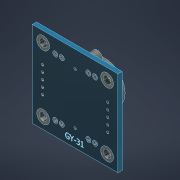
# Autodesk Inventor part: Color_sensor_PCB
Saved by Autodesk Inventor 2021 (Build 250183000, 183)
## iProperties
Created: 2016-09-21
Part Number: Color_sensor_PCB
Material: ABS Plastic
Document SubType Name: Modeling
Designer: Ádi
Density: 1.06 g/cm^3
Appearance: Sky Blue Medium
Author: Ádi
Autodesk Inventor part; units mm, degrees
(part 1 of 2)
ref_plane "YZ Plane" through (0, 0, 0) normal (1, 0, 0) x (0, 1, 0)
ref_plane "XZ Plane" through (0, 0, 0) normal (0, 1, 0) x (-1, 0, 0)
ref_plane "XY Plane" through (0, 0, 0) normal (0, 0, 1) x (1, 0, 0)
sketch "Sketch1" plane through (0, 0, 0) normal (0, 1, 0) x (-1, 0, 0)
  line L0 (-16.75, 16.75) -> (16.75, 16.75)
  line L1 (16.75, 16.75) -> (16.75, -16.75)
  line L2 (16.75, -16.75) -> (-16.75, -16.75)
  line L3 (-16.75, -16.75) -> (-16.75, 16.75)
  line L4 (-16.75, 16.75) -> (16.75, -16.75) construction
  line L5 (16.75, 16.75) -> (-16.75, -16.75) construction
  point P0 (0, 0)
  dimension "d0" = 33.5
  dimension "d1" = 33.5
  constraints: 12 end point, 2 midpoint, 2 parallel, 1 horizontal, 1 perpendicular
  measures "d0" distance of L1.end L2.end
  measures "d1" distance of L0.end L1.end
extrude "Extrusion1" add sketch "Sketch1" along normal blind 1.65
sketch "Sketch2" plane through (0, 1.65, 0) normal (0, 1, 0) x (1, 0, 0)
  line L0 (16.75, -16.75) -> (16.75, 16.75) projected
  line L1 (-16.75, -16.75) -> (16.75, -16.75) projected
  point P0 (0, 0)
  point P1 (-12.4997, -12.6164)
  point P2 (-12.4997, 12.3836)
  point P3 (12.5, 12.5)
  point P4 (12.5, -12.5)
  dimension "d4" = 25
  dimension "d5" = 25
  dimension "d6" = 25
  dimension "d7" = 25
  dimension "d8" = 0
  dimension "d9" = 4.25
  dimension "d10" = 4.25
  measures "d4" distance of point (12.5, 12.5) point (12.5, -12.5)
  measures "d5" distance of point (-12.5, 12.384) point (12.5, 12.5)
  measures "d6" distance of point (-12.5, -12.616) point (-12.5, 12.384)
  measures "d7" distance of point (12.5, -12.5) point (-12.5, -12.616)
  measures "d8" horizontal distance of point (12.5, 12.5) point (12.5, -12.5)
  measures "d9" distance from line of L0 point (12.5, -12.5)
  measures "d10" distance from line of point (12.5, -12.5) L1
hole "Hole1" at (-12.4997, 1.65, 12.6164) at (-12.4997, 1.65, -12.3836) at (12.5, 1.65, -12.5) at (12.5, 1.65, 12.5) direction (0, -1, 0) diameter 3 depth 8 tip angle 118
sketch "Sketch3" plane through (0, 1.65, 0) normal (0, 1, 0) x (1, 0, 0)
  circle A0 centre (12.5, 12.5) radius 1.5 projected
  circle A1 centre (-12.4997, -12.6164) radius 1.5 projected
  circle A2 centre (-12.4997, 12.3836) radius 1.5 projected
  circle A3 centre (12.5, -12.5) radius 1.5 projected
  line L0 (-16.75, -16.75) -> (16.75, -16.75) projected
  line L1 (16.75, -16.75) -> (16.75, 16.75) projected
  line L2 (16.75, 16.75) -> (-16.75, 16.75) projected
  line L3 (-16.75, 16.75) -> (-16.75, -16.75) projected
  circle A4 centre (-12.4997, -12.6164) radius 1.5 projected
  circle A5 centre (-12.4997, -12.6164) radius 2.5
  circle A6 centre (-12.4997, 12.3836) radius 2.5
  circle A7 centre (12.5, 12.5) radius 2.5
  circle A8 centre (12.5, -12.5) radius 1.5 projected
  circle A9 centre (12.5, -12.5) radius 2.5
  point P0 (0, 0)
  dimension "d18" = 5
  dimension "d19" = 5
  dimension "d20" = 5
  dimension "d21" = 5
  constraints: 4 centre point, 4 coincident
  measures "d18" diameter of A5
  measures "d19" diameter of A6
  measures "d20" diameter of A7
  measures "d21" diameter of A9
extrude "Extrusion2" add sketch "Sketch3" along normal blind 0.01 contours A5 | A6 | A7 | A9
sketch "Sketch4" plane through (0, 0, 0) normal (0, -1, 0) x (1, 0, 0)
  circle A0 centre (12.5, -12.5) radius 1.5 projected
  circle A1 centre (-12.4997, 12.6164) radius 1.5 projected
  circle A2 centre (-12.4997, -12.3836) radius 1.5 projected
  circle A3 centre (12.5, 12.5) radius 1.5 projected
  line L0 (16.75, 16.75) -> (-16.75, 16.75) projected
  line L1 (-16.75, 16.75) -> (-16.75, -16.75) projected
  line L2 (-16.75, -16.75) -> (16.75, -16.75) projected
  line L3 (16.75, -16.75) -> (16.75, 16.75) projected
  circle A4 centre (12.5, 12.5) radius 2.5 projected
  circle A5 centre (12.5, 12.5) radius 2.5
  circle A6 centre (12.5, -12.5) radius 2.5
  circle A7 centre (-12.4997, -12.3836) radius 2.5
  circle A8 centre (-12.4997, 12.6164) radius 2.5
  point P0 (0, 0)
  constraints: 4 centre point, 4 coincident
extrude "Extrusion3" add sketch "Sketch4" along normal blind 0.01 contours A4 | A6 | A7 | A8
sketch "Sketch5" plane through (0, 0, 0) normal (0, -1, 0) x (1, 0, 0)
  line L0 (16.75, -16.75) -> (16.75, 16.75) projected
  line L1 (16.75, -16.75) -> (-16.75, -16.75) projected
  point P0 (0, 0)
  point P1 (12.75, -5.07)
  point P2 (12.75, -2.53)
  point P3 (12.75, 0.01)
  point P4 (12.75, 2.55)
  point P5 (12.75, 5.09)
  dimension "d26" = 4
  dimension "d29" = 2.54
  dimension "d41" = 11.68
  constraints: 1 vertical, 4 other
  measures "d26" distance from line of point (12.75, -5.07) L0
  measures "d29" distance of point (12.75, -5.07) point (12.75, -2.53)
  measures "d41" distance from line of L1 point (12.75, -5.07)
hole "Hole2" at (12.75, 0, -5.07) at (12.75, 0, -2.53) at (12.75, 0, 0.01) at (12.75, 0, 2.55) at (12.75, 0, 5.09) direction (0, 1, 0) diameter 1 depth 8 tip angle 118
mirror "Mirror1" about plane through (0, 0, 0) normal (1, 0, 0) of "Hole2"
sketch "Sketch6" plane through (0, 1.65, 0) normal (0, 1, 0) x (1, 0, 0)
  circle A0 centre (-12.75, -2.55) radius 0.5 projected
  circle A1 centre (-12.75, 2.53) radius 0.5 projected
  circle A2 centre (-12.75, 5.07) radius 0.5 projected
  circle A3 centre (-12.75, -0.01) radius 0.5 projected
  circle A4 centre (-12.75, -5.09) radius 0.5 projected
  circle A5 centre (12.75, -2.55) radius 0.5 projected
  circle A6 centre (12.75, 2.53) radius 0.5 projected
  circle A7 centre (12.75, 5.07) radius 0.5 projected
  circle A8 centre (12.75, -0.01) radius 0.5 projected
  circle A9 centre (12.75, -5.09) radius 0.5 projected
  circle A10 centre (12.5, 12.5) radius 2.5 projected
  circle A11 centre (-12.4997, -12.6164) radius 2.5 projected
  circle A12 centre (-12.4997, 12.3836) radius 2.5 projected
  circle A13 centre (12.5, -12.5) radius 2.5 projected
  line L0 (-16.75, -16.75) -> (16.75, -16.75) projected
  line L1 (16.75, -16.75) -> (16.75, 16.75) projected
  line L2 (16.75, 16.75) -> (-16.75, 16.75) projected
  line L3 (-16.75, 16.75) -> (-16.75, -16.75) projected
  circle A14 centre (12.75, 5.07) radius 0.5 projected
  circle A15 centre (12.75, 5.07) radius 1
  circle A16 centre (12.75, 2.53) radius 0.5 projected
  circle A17 centre (12.75, 2.53) radius 1
  circle A18 centre (12.75, -0.01) radius 0.5 projected
  circle A19 centre (12.75, -0.01) radius 1
  circle A20 centre (12.75, -2.55) radius 1
  circle A21 centre (12.75, -5.09) radius 1
  point P0 (0, 0)
  dimension "d42" = 2
  dimension "d43" = 2
  dimension "d44" = 2
  dimension "d45" = 2
  dimension "d46" = 2
  constraints: 5 centre point, 5 coincident
  measures "d42" diameter of A15
  measures "d43" diameter of A17
  measures "d44" diameter of A19
  measures "d45" diameter of A20
  measures "d46" diameter of A21
extrude "Extrusion4" add sketch "Sketch6" along normal blind 0.01 contours A15 | A17 | A19 | A20 | A21
mirror "Mirror2" about plane through (0, 0, 0) normal (1, 0, 0) of "Extrusion4"
sketch "Sketch7" plane through (0, 1.65, 0) normal (0, 1, 0) x (1, 0, 0)
  line L0 (14.4, -6.51) -> (11.1, -6.51)
  line L1 (11.1, -6.51) -> (11.1, 6.49)
  line L2 (11.1, 6.49) -> (14.4, 6.49)
  line L3 (14.4, 6.49) -> (14.4, -6.51)
  circle A0 centre (12.75, -0.01) radius 0.5 projected
  line L4 (14.4, -6.51) -> (11.1, 6.49) construction
  line L5 (11.1, -6.51) -> (14.4, 6.49) construction
  line L6 (14, 6.09) -> (11.5, 6.09)
  line L7 (11.5, 6.09) -> (11.5, -6.11)
  line L8 (11.5, -6.11) -> (14, -6.11)
  line L9 (14, -6.11) -> (14, 6.09)
  line L10 (14, 6.09) -> (11.5, -6.11) construction
  line L11 (11.5, 6.09) -> (14, -6.11) construction
  point P0 (0, 0)
  dimension "d49" = 3.3
  dimension "d50" = 13
  dimension "d51" = 0.4
  dimension "d52" = 0.4
  constraints: 24 end point, 4 midpoint, 4 parallel, 2 horizontal, 2 perpendicular
  measures "d49" distance of L1.end L2.end
  measures "d50" distance between parallel lines of L2 L0
  measures "d51" distance between parallel lines of L8 L0
  measures "d52" distance between parallel lines of L1 L7
extrude "Extrusion5" add sketch "Sketch7" along normal blind 0.01 contours L0 L1 L2 L3
mirror "Mirror3" about plane through (0, 0, 0) normal (1, 0, 0) of "Extrusion5"
sketch "Sketch8" plane through (0, 1.65, 0) normal (0, 1, 0) x (1, 0, 0)
  line L0 (14.9046, -7.6087) -> (14.9046, 13.5384) construction
  line L1 (14.9046, 13.5384) -> (16.4666, 13.5384) construction
  line L2 (16.4666, 13.5384) -> (16.4666, -7.6087) construction
  line L3 (16.4666, -7.6087) -> (14.9046, -7.6087) construction
  line L4 (-14.8755, 8.2478) -> (-14.8755, -7.59) construction
  line L5 (-14.8755, -7.59) -> (-16.1781, -7.59) construction
  line L6 (-16.1781, -7.59) -> (-16.1781, 8.2478) construction
  line L7 (-16.1781, 8.2478) -> (-14.8755, 8.2478) construction
  line L8 (14.93, -6.5754) -> (16.18, -7.0059)
  line L9 (16.18, -7.0059) -> (16.18, -7.1852)
  line L10 (16.18, -7.1852) -> (14.93, -7.6157)
  line L11 (14.93, -7.6157) -> (14.93, -7.4375)
  line L12 (14.93, -7.4375) -> (15.9682, -7.091)
  line L13 (15.9682, -7.091) -> (14.93, -6.7446)
  line L14 (14.93, -6.7446) -> (14.93, -6.5754)
  spline S0 degree 2 poles (16.2022, -5.9677) (16.2022, -6.0892) (16.1202, -6.2948) (16.0381, -6.3698) knots 0 0 0 1 2 2 2
  spline S1 degree 2 poles (16.0381, -6.3698) (15.9571, -6.4448) (15.714, -6.5268) (15.556, -6.5268) knots 0 0 0 1 2 2 2
  spline S2 degree 2 poles (15.556, -6.5268) (15.399, -6.5268) (15.166, -6.4468) (15.0799, -6.3708) knots 0 0 0 1 2 2 2
  spline S3 degree 2 poles (15.0799, -6.3708) (14.9958, -6.2959) (14.9077, -6.0912) (14.9077, -5.9646) knots 0 0 0 1 2 2 2
  spline S4 degree 2 poles (14.9077, -5.9646) (14.9077, -5.9018) (14.9259, -5.7914) (14.9401, -5.7448) knots 0 0 0 1 2 2 2
  spline S5 degree 2 poles (14.9401, -5.7448) (14.9533, -5.7043) (14.9907, -5.6202) (15.013, -5.5787) knots 0 0 0 1 2 2 2
  line L15 (15.013, -5.5787) -> (15.2136, -5.5787)
  line L16 (15.2136, -5.5787) -> (15.2136, -5.5918)
  spline S6 degree 2 poles (15.2136, -5.5918) (15.1933, -5.6141) (15.1366, -5.683) (15.1093, -5.7326) knots 0 0 0 1 2 2 2
  spline S7 degree 2 poles (15.1093, -5.7326) (15.0829, -5.7803) (15.0495, -5.8927) (15.0495, -5.9656) knots 0 0 0 1 2 2 2
  spline S8 degree 2 poles (15.0495, -5.9656) (15.0495, -6.0456) (15.1153, -6.1885) (15.1781, -6.2422) knots 0 0 0 1 2 2 2
  spline S9 degree 2 poles (15.1781, -6.2422) (15.242, -6.2948) (15.4354, -6.3536) (15.556, -6.3536) knots 0 0 0 1 2 2 2
  spline S10 degree 2 poles (15.556, -6.3536) (15.6846, -6.3536) (15.87, -6.2918) (15.9338, -6.2381) knots 0 0 0 1 2 2 2
  spline S11 degree 2 poles (15.9338, -6.2381) (15.9956, -6.1854) (16.0584, -6.0446) (16.0584, -5.9656) knots 0 0 0 1 2 2 2
  spline S12 degree 2 poles (16.0584, -5.9656) (16.0584, -5.8937) (16.0229, -5.7711) (15.9966, -5.7235) knots 0 0 0 1 2 2 2
  spline S13 degree 2 poles (15.9966, -5.7235) (15.9703, -5.6779) (15.9156, -5.6101) (15.8963, -5.5908) knots 0 0 0 1 2 2 2
  line L17 (15.8963, -5.5908) -> (15.8963, -5.5787)
  line L18 (15.8963, -5.5787) -> (16.0949, -5.5787)
  spline S14 degree 2 poles (16.0949, -5.5787) (16.1141, -5.6202) (16.1496, -5.6931) (16.1658, -5.7448) knots 0 0 0 1 2 2 2
  spline S15 degree 2 poles (16.1658, -5.7448) (16.184, -5.7995) (16.2022, -5.8927) (16.2022, -5.9677) knots 0 0 0 1 2 2 2
  spline S16 degree 2 poles (16.2022, -4.9354) (16.2022, -5.057) (16.1202, -5.2626) (16.0381, -5.3376) knots 0 0 0 1 2 2 2
  spline S17 degree 2 poles (16.0381, -5.3376) (15.9571, -5.4125) (15.714, -5.4946) (15.556, -5.4946) knots 0 0 0 1 2 2 2
  spline S18 degree 2 poles (15.556, -5.4946) (15.399, -5.4946) (15.166, -5.4146) (15.0799, -5.3386) knots 0 0 0 1 2 2 2
  spline S19 degree 2 poles (15.0799, -5.3386) (14.9958, -5.2636) (14.9077, -5.059) (14.9077, -4.9324) knots 0 0 0 1 2 2 2
  spline S20 degree 2 poles (14.9077, -4.9324) (14.9077, -4.8696) (14.9259, -4.7592) (14.9401, -4.7126) knots 0 0 0 1 2 2 2
  spline S21 degree 2 poles (14.9401, -4.7126) (14.9533, -4.6721) (14.9907, -4.588) (15.013, -4.5465) knots 0 0 0 1 2 2 2
  line L19 (15.013, -4.5465) -> (15.2136, -4.5465)
  line L20 (15.2136, -4.5465) -> (15.2136, -4.5596)
  spline S22 degree 2 poles (15.2136, -4.5596) (15.1933, -4.5819) (15.1366, -4.6508) (15.1093, -4.7004) knots 0 0 0 1 2 2 2
  spline S23 degree 2 poles (15.1093, -4.7004) (15.0829, -4.748) (15.0495, -4.8605) (15.0495, -4.9334) knots 0 0 0 1 2 2 2
  spline S24 degree 2 poles (15.0495, -4.9334) (15.0495, -5.0134) (15.1153, -5.1563) (15.1781, -5.21) knots 0 0 0 1 2 2 2
  spline S25 degree 2 poles (15.1781, -5.21) (15.242, -5.2626) (15.4354, -5.3214) (15.556, -5.3214) knots 0 0 0 1 2 2 2
  spline S26 degree 2 poles (15.556, -5.3214) (15.6846, -5.3214) (15.87, -5.2596) (15.9338, -5.2059) knots 0 0 0 1 2 2 2
  spline S27 degree 2 poles (15.9338, -5.2059) (15.9956, -5.1532) (16.0584, -5.0124) (16.0584, -4.9334) knots 0 0 0 1 2 2 2
  spline S28 degree 2 poles (16.0584, -4.9334) (16.0584, -4.8615) (16.0229, -4.7389) (15.9966, -4.6913) knots 0 0 0 1 2 2 2
  spline S29 degree 2 poles (15.9966, -4.6913) (15.9703, -4.6457) (15.9156, -4.5779) (15.8963, -4.5586) knots 0 0 0 1 2 2 2
  line L21 (15.8963, -4.5586) -> (15.8963, -4.5465)
  line L22 (15.8963, -4.5465) -> (16.0949, -4.5465)
  spline S30 degree 2 poles (16.0949, -4.5465) (16.1141, -4.588) (16.1496, -4.6609) (16.1658, -4.7126) knots 0 0 0 1 2 2 2
  spline S31 degree 2 poles (16.1658, -4.7126) (16.184, -4.7673) (16.2022, -4.8605) (16.2022, -4.9354) knots 0 0 0 1 2 2 2
  spline S32 degree 2 poles (16.2022, -3.5061) (16.2022, -3.6419) (16.1455, -3.8323) (16.105, -3.9164) knots 0 0 0 1 2 2 2
  line L23 (16.105, -3.9164) -> (15.8963, -3.9164)
  line L24 (15.8963, -3.9164) -> (15.8963, -3.9042)
  spline S33 degree 2 poles (15.8963, -3.9042) (15.9733, -3.8222) (16.0584, -3.6145) (16.0584, -3.5183) knots 0 0 0 1 2 2 2
  spline S34 degree 2 poles (16.0584, -3.5183) (16.0584, -3.3805) (15.9439, -3.2397) (15.8497, -3.2397) knots 0 0 0 1 2 2 2
  spline S35 degree 2 poles (15.8497, -3.2397) (15.7748, -3.2397) (15.6816, -3.3137) (15.6583, -3.3937) knots 0 0 0 1 2 2 2
  spline S36 degree 2 poles (15.6583, -3.3937) (15.6421, -3.4514) (15.6198, -3.5477) (15.6016, -3.6196) knots 0 0 0 1 2 2 2
  spline S37 degree 2 poles (15.6016, -3.6196) (15.5843, -3.6844) (15.5327, -3.7867) (15.4911, -3.8262) knots 0 0 0 1 2 2 2
  spline S38 degree 2 poles (15.4911, -3.8262) (15.4496, -3.8647) (15.3382, -3.9073) (15.2652, -3.9073) knots 0 0 0 1 2 2 2
  spline S39 degree 2 poles (15.2652, -3.9073) (15.1133, -3.9073) (14.9077, -3.6702) (14.9077, -3.4869) knots 0 0 0 1 2 2 2
  spline S40 degree 2 poles (14.9077, -3.4869) (14.9077, -3.3815) (14.9492, -3.1952) (14.9887, -3.1151) knots 0 0 0 1 2 2 2
  line L25 (14.9887, -3.1151) -> (15.1873, -3.1151)
  line L26 (15.1873, -3.1151) -> (15.1873, -3.1273)
  spline S41 degree 2 poles (15.1873, -3.1273) (15.1326, -3.1871) (15.0515, -3.3734) (15.0515, -3.4758) knots 0 0 0 1 2 2 2
  spline S42 degree 2 poles (15.0515, -3.4758) (15.0515, -3.5912) (15.1599, -3.7341) (15.248, -3.7341) knots 0 0 0 1 2 2 2
  spline S43 degree 2 poles (15.248, -3.7341) (15.327, -3.7341) (15.4212, -3.65) (15.4425, -3.571) knots 0 0 0 1 2 2 2
  spline S44 degree 2 poles (15.4425, -3.571) (15.4567, -3.5183) (15.4932, -3.3653) (15.5084, -3.3147) knots 0 0 0 1 2 2 2
  spline S45 degree 2 poles (15.5084, -3.3147) (15.5479, -3.186) (15.7069, -3.0665) (15.8234, -3.0665) knots 0 0 0 1 2 2 2
  spline S46 degree 2 poles (15.8234, -3.0665) (15.8973, -3.0665) (16.0392, -3.1263) (16.0888, -3.18) knots 0 0 0 1 2 2 2
  spline S47 degree 2 poles (16.0888, -3.18) (16.1435, -3.2397) (16.2022, -3.3917) (16.2022, -3.5061) knots 0 0 0 1 2 2 2
  line L27 (16.18, -2.2247) -> (16.18, -2.8345)
  line L28 (16.18, -2.8345) -> (16.0523, -2.8345)
  line L29 (16.0523, -2.8345) -> (16.0523, -2.6076)
  line L30 (16.0523, -2.6076) -> (15.2146, -2.6076)
  line L31 (15.2146, -2.6076) -> (15.2146, -2.8345)
  line L32 (15.2146, -2.8345) -> (15.1001, -2.8345)
  spline S48 degree 2 poles (15.1001, -2.8345) (15.1001, -2.7059) (15.0272, -2.5843) (14.9259, -2.5762) knots 0 0 0 1 2 2 2
  line L33 (14.9259, -2.5762) -> (14.9259, -2.4466)
  line L34 (14.9259, -2.4466) -> (16.0523, -2.4466)
  line L35 (16.0523, -2.4466) -> (16.0523, -2.2247)
  line L36 (16.0523, -2.2247) -> (16.18, -2.2247)
  spline S49 degree 2 poles (16.2022, -1.074) (16.2022, -1.2097) (16.1455, -1.4002) (16.105, -1.4843) knots 0 0 0 1 2 2 2
  line L37 (16.105, -1.4843) -> (15.8963, -1.4843)
  line L38 (15.8963, -1.4843) -> (15.8963, -1.4721)
  spline S50 degree 2 poles (15.8963, -1.4721) (15.9733, -1.3901) (16.0584, -1.1824) (16.0584, -1.0862) knots 0 0 0 1 2 2 2
  spline S51 degree 2 poles (16.0584, -1.0862) (16.0584, -0.9484) (15.9439, -0.8076) (15.8497, -0.8076) knots 0 0 0 1 2 2 2
  spline S52 degree 2 poles (15.8497, -0.8076) (15.7748, -0.8076) (15.6816, -0.8815) (15.6583, -0.9616) knots 0 0 0 1 2 2 2
  spline S53 degree 2 poles (15.6583, -0.9616) (15.6421, -1.0193) (15.6198, -1.1155) (15.6016, -1.1875) knots 0 0 0 1 2 2 2
  spline S54 degree 2 poles (15.6016, -1.1875) (15.5843, -1.2523) (15.5327, -1.3546) (15.4911, -1.3941) knots 0 0 0 1 2 2 2
  spline S55 degree 2 poles (15.4911, -1.3941) (15.4496, -1.4326) (15.3382, -1.4751) (15.2652, -1.4751) knots 0 0 0 1 2 2 2
  spline S56 degree 2 poles (15.2652, -1.4751) (15.1133, -1.4751) (14.9077, -1.2381) (14.9077, -1.0548) knots 0 0 0 1 2 2 2
  spline S57 degree 2 poles (14.9077, -1.0548) (14.9077, -0.9494) (14.9492, -0.763) (14.9887, -0.683) knots 0 0 0 1 2 2 2
  line L39 (14.9887, -0.683) -> (15.1873, -0.683)
  line L40 (15.1873, -0.683) -> (15.1873, -0.6952)
  spline S58 degree 2 poles (15.1873, -0.6952) (15.1326, -0.7549) (15.0515, -0.9413) (15.0515, -1.0436) knots 0 0 0 1 2 2 2
  spline S59 degree 2 poles (15.0515, -1.0436) (15.0515, -1.1591) (15.1599, -1.3019) (15.248, -1.3019) knots 0 0 0 1 2 2 2
  spline S60 degree 2 poles (15.248, -1.3019) (15.327, -1.3019) (15.4212, -1.2179) (15.4425, -1.1388) knots 0 0 0 1 2 2 2
  spline S61 degree 2 poles (15.4425, -1.1388) (15.4567, -1.0862) (15.4932, -0.9332) (15.5084, -0.8826) knots 0 0 0 1 2 2 2
  spline S62 degree 2 poles (15.5084, -0.8826) (15.5479, -0.7539) (15.7069, -0.6344) (15.8234, -0.6344) knots 0 0 0 1 2 2 2
  spline S63 degree 2 poles (15.8234, -0.6344) (15.8973, -0.6344) (16.0392, -0.6941) (16.0888, -0.7478) knots 0 0 0 1 2 2 2
  spline S64 degree 2 poles (16.0888, -0.7478) (16.1435, -0.8076) (16.2022, -0.9595) (16.2022, -1.074) knots 0 0 0 1 2 2 2
  spline S65 degree 2 poles (15.555, 0.2773) (15.8913, 0.2773) (16.2063, 0.0818) (16.2063, -0.1218) knots 0 0 0 1 2 2 2
  spline S66 degree 2 poles (16.2063, -0.1218) (16.2063, -0.3285) (15.8852, -0.5219) (15.556, -0.5219) knots 0 0 0 1 2 2 2
  spline S67 degree 2 poles (15.556, -0.5219) (15.2176, -0.5219) (14.9046, -0.3264) (14.9046, -0.1218) knots 0 0 0 1 2 2 2
  spline S68 degree 2 poles (14.9046, -0.1218) (14.9046, 0.0838) (15.2288, 0.2773) (15.555, 0.2773) knots 0 0 0 1 2 2 2
  spline S69 degree 2 poles (15.9358, 0.0625) (15.874, 0.0868) (15.6836, 0.1071) (15.555, 0.1071) knots 0 0 0 1 2 2 2
  spline S70 degree 2 poles (15.555, 0.1071) (15.4263, 0.1071) (15.2369, 0.0868) (15.1731, 0.0615) knots 0 0 0 1 2 2 2
  spline S71 degree 2 poles (15.1731, 0.0615) (15.1093, 0.0362) (15.0434, -0.0519) (15.0434, -0.1218) knots 0 0 0 1 2 2 2
  spline S72 degree 2 poles (15.0434, -0.1218) (15.0434, -0.1917) (15.1093, -0.2819) (15.1751, -0.3082) knots 0 0 0 1 2 2 2
  spline S73 degree 2 poles (15.1751, -0.3082) (15.2389, -0.3335) (15.4334, -0.3518) (15.556, -0.3518) knots 0 0 0 1 2 2 2
  spline S74 degree 2 poles (15.556, -0.3518) (15.6877, -0.3518) (15.8639, -0.3356) (15.9328, -0.3092) knots 0 0 0 1 2 2 2
  spline S75 degree 2 poles (15.9328, -0.3092) (15.9976, -0.2849) (16.0675, -0.1948) (16.0675, -0.1218) knots 0 0 0 1 2 2 2
  spline S76 degree 2 poles (16.0675, -0.1218) (16.0675, -0.0529) (16.0017, 0.0372) (15.9358, 0.0625) knots 0 0 0 1 2 2 2
  line L41 (16.18, 1.7339) -> (16.18, 1.0097)
  line L42 (16.18, 1.0097) -> (14.93, 1.0097)
  line L43 (14.93, 1.0097) -> (14.93, 1.1758)
  line L44 (14.93, 1.1758) -> (16.0321, 1.1758)
  line L45 (16.0321, 1.1758) -> (16.0321, 1.7339)
  line L46 (16.0321, 1.7339) -> (16.18, 1.7339)
  line L47 (16.18, 1.8646) -> (14.93, 1.8646)
  line L48 (14.93, 1.8646) -> (14.93, 2.6466)
  line L49 (14.93, 2.6466) -> (15.0779, 2.6466)
  line L50 (15.0779, 2.6466) -> (15.0779, 2.0307)
  line L51 (15.0779, 2.0307) -> (15.4202, 2.0307)
  line L52 (15.4202, 2.0307) -> (15.4202, 2.6051)
  line L53 (15.4202, 2.6051) -> (15.5681, 2.6051)
  line L54 (15.5681, 2.6051) -> (15.5681, 2.0307)
  line L55 (15.5681, 2.0307) -> (16.0321, 2.0307)
  line L56 (16.0321, 2.0307) -> (16.0321, 2.6466)
  line L57 (16.0321, 2.6466) -> (16.18, 2.6466)
  line L58 (16.18, 2.6466) -> (16.18, 1.8646)
  spline S77 degree 2 poles (15.556, 3.8146) (15.7272, 3.8146) (16.0027, 3.6758) (16.0797, 3.5593) knots 0 0 0 1 2 2 2
  spline S78 degree 2 poles (16.0797, 3.5593) (16.1394, 3.4641) (16.18, 3.2686) (16.18, 3.1166) knots 0 0 0 1 2 2 2
  line L59 (16.18, 3.1166) -> (16.18, 2.8289)
  line L60 (16.18, 2.8289) -> (14.93, 2.8289)
  line L61 (14.93, 2.8289) -> (14.93, 3.1136)
  spline S79 degree 2 poles (14.93, 3.1136) (14.93, 3.2898) (14.9826, 3.4904) (15.0292, 3.5613) knots 0 0 0 1 2 2 2
  spline S80 degree 2 poles (15.0292, 3.5613) (15.1093, 3.6819) (15.3736, 3.8146) (15.556, 3.8146) knots 0 0 0 1 2 2 2
  spline S81 degree 2 poles (15.5539, 3.6413) (15.4101, 3.6413) (15.2065, 3.5461) (15.1488, 3.4519) knots 0 0 0 1 2 2 2
  spline S82 degree 2 poles (15.1488, 3.4519) (15.1093, 3.3851) (15.0738, 3.2341) (15.0738, 3.1217) knots 0 0 0 1 2 2 2
  line L62 (15.0738, 3.1217) -> (15.0738, 2.9951)
  line L63 (15.0738, 2.9951) -> (16.0361, 2.9951)
  line L64 (16.0361, 2.9951) -> (16.0361, 3.1217)
  spline S83 degree 2 poles (16.0361, 3.1217) (16.0361, 3.2321) (16.0007, 3.3992) (15.9531, 3.4671) knots 0 0 0 1 2 2 2
  spline S84 degree 2 poles (15.9531, 3.4671) (15.8943, 3.5542) (15.6998, 3.6413) (15.5539, 3.6413) knots 0 0 0 1 2 2 2
  spline S85 degree 2 poles (16.2043, 5.0554) (16.2043, 4.9227) (16.1232, 4.7029) (16.0412, 4.6239) knots 0 0 0 1 2 2 2
  spline S86 degree 2 poles (16.0412, 4.6239) (15.9581, 4.5449) (15.713, 4.4608) (15.5539, 4.4608) knots 0 0 0 1 2 2 2
  spline S87 degree 2 poles (15.5539, 4.4608) (15.403, 4.4608) (15.164, 4.5459) (15.0789, 4.6249) knots 0 0 0 1 2 2 2
  spline S88 degree 2 poles (15.0789, 4.6249) (14.9968, 4.7009) (14.9077, 4.9238) (14.9077, 5.0565) knots 0 0 0 1 2 2 2
  spline S89 degree 2 poles (14.9077, 5.0565) (14.9077, 5.1203) (14.9259, 5.2358) (14.9421, 5.2884) knots 0 0 0 1 2 2 2
  spline S90 degree 2 poles (14.9421, 5.2884) (14.9543, 5.331) (14.9988, 5.4343) (15.015, 5.4657) knots 0 0 0 1 2 2 2
  line L65 (15.015, 5.4657) -> (15.2156, 5.4657)
  line L66 (15.2156, 5.4657) -> (15.2156, 5.4515)
  spline S91 degree 2 poles (15.2156, 5.4515) (15.1883, 5.4201) (15.1386, 5.3543) (15.1103, 5.2935) knots 0 0 0 1 2 2 2
  spline S92 degree 2 poles (15.1103, 5.2935) (15.0849, 5.2428) (15.0515, 5.1122) (15.0515, 5.0372) knots 0 0 0 1 2 2 2
  spline S93 degree 2 poles (15.0515, 5.0372) (15.0515, 4.8569) (15.323, 4.6341) (15.5489, 4.6341) knots 0 0 0 1 2 2 2
  spline S94 degree 2 poles (15.5489, 4.6341) (15.6745, 4.6341) (15.8629, 4.6928) (15.9277, 4.7485) knots 0 0 0 1 2 2 2
  spline S95 degree 2 poles (15.9277, 4.7485) (15.9926, 4.8022) (16.0604, 4.9541) (16.0604, 5.0494) knots 0 0 0 1 2 2 2
  spline S96 degree 2 poles (16.0604, 5.0494) (16.0604, 5.1193) (16.0402, 5.2591) (16.0199, 5.3067) knots 0 0 0 1 2 2 2
  line L67 (16.0199, 5.3067) -> (15.6968, 5.3067)
  line L68 (15.6968, 5.3067) -> (15.6968, 5.017)
  line L69 (15.6968, 5.017) -> (15.5509, 5.017)
  line L70 (15.5509, 5.017) -> (15.5509, 5.4708)
  line L71 (15.5509, 5.4708) -> (16.0969, 5.4708)
  spline S97 degree 2 poles (16.0969, 5.4708) (16.1111, 5.4394) (16.1546, 5.332) (16.1678, 5.2864) knots 0 0 0 1 2 2 2
  spline S98 degree 2 poles (16.1678, 5.2864) (16.186, 5.2246) (16.2043, 5.1253) (16.2043, 5.0554) knots 0 0 0 1 2 2 2
  line L72 (16.18, 6.5739) -> (16.18, 6.3875)
  line L73 (16.18, 6.3875) -> (15.1022, 5.8344)
  line L74 (15.1022, 5.8344) -> (16.18, 5.8344)
  line L75 (16.18, 5.8344) -> (16.18, 5.6794)
  line L76 (16.18, 5.6794) -> (14.93, 5.6794)
  line L77 (14.93, 5.6794) -> (14.93, 5.9155)
  line L78 (14.93, 5.9155) -> (15.9196, 6.4189)
  line L79 (15.9196, 6.4189) -> (14.93, 6.4189)
  line L80 (14.93, 6.4189) -> (14.93, 6.5739)
  line L81 (14.93, 6.5739) -> (16.18, 6.5739)
  spline S99 degree 2 poles (15.556, 7.8127) (15.7272, 7.8127) (16.0027, 7.674) (16.0797, 7.5575) knots 0 0 0 1 2 2 2
  spline S100 degree 2 poles (16.0797, 7.5575) (16.1394, 7.4623) (16.18, 7.2667) (16.18, 7.1148) knots 0 0 0 1 2 2 2
  line L82 (16.18, 7.1148) -> (16.18, 6.8271)
  line L83 (16.18, 6.8271) -> (14.93, 6.8271)
  line L84 (14.93, 6.8271) -> (14.93, 7.1118)
  spline S101 degree 2 poles (14.93, 7.1118) (14.93, 7.288) (14.9826, 7.4886) (15.0292, 7.5595) knots 0 0 0 1 2 2 2
  spline S102 degree 2 poles (15.0292, 7.5595) (15.1093, 7.68) (15.3736, 7.8127) (15.556, 7.8127) knots 0 0 0 1 2 2 2
  spline S103 degree 2 poles (15.5539, 7.6395) (15.4101, 7.6395) (15.2065, 7.5443) (15.1488, 7.4501) knots 0 0 0 1 2 2 2
  spline S104 degree 2 poles (15.1488, 7.4501) (15.1093, 7.3832) (15.0738, 7.2323) (15.0738, 7.1199) knots 0 0 0 1 2 2 2
  line L85 (15.0738, 7.1199) -> (15.0738, 6.9932)
  line L86 (15.0738, 6.9932) -> (16.0361, 6.9932)
  line L87 (16.0361, 6.9932) -> (16.0361, 7.1199)
  spline S105 degree 2 poles (16.0361, 7.1199) (16.0361, 7.2303) (16.0007, 7.3974) (15.9531, 7.4653) knots 0 0 0 1 2 2 2
  spline S106 degree 2 poles (15.9531, 7.4653) (15.8943, 7.5524) (15.6998, 7.6395) (15.5539, 7.6395) knots 0 0 0 1 2 2 2
  spline S107 degree 2 poles (-16.1761, 7.5974) (-16.1761, 7.7301) (-16.0951, 7.9499) (-16.013, 8.029) knots 0 0 0 1 2 2 2
  spline S108 degree 2 poles (-16.013, 8.029) (-15.93, 8.108) (-15.6848, 8.192) (-15.5258, 8.192) knots 0 0 0 1 2 2 2
  spline S109 degree 2 poles (-15.5258, 8.192) (-15.3749, 8.192) (-15.1358, 8.107) (-15.0507, 8.0279) knots 0 0 0 1 2 2 2
  spline S110 degree 2 poles (-15.0507, 8.0279) (-14.9687, 7.952) (-14.8795, 7.7291) (-14.8795, 7.5964) knots 0 0 0 1 2 2 2
  spline S111 degree 2 poles (-14.8795, 7.5964) (-14.8795, 7.5326) (-14.8978, 7.4171) (-14.914, 7.3645) knots 0 0 0 1 2 2 2
  spline S112 degree 2 poles (-14.914, 7.3645) (-14.9261, 7.3219) (-14.9707, 7.2186) (-14.9869, 7.1872) knots 0 0 0 1 2 2 2
  line L88 (-14.9869, 7.1872) -> (-15.1875, 7.1872)
  line L89 (-15.1875, 7.1872) -> (-15.1875, 7.2014)
  spline S113 degree 2 poles (-15.1875, 7.2014) (-15.1601, 7.2328) (-15.1105, 7.2986) (-15.0821, 7.3594) knots 0 0 0 1 2 2 2
  spline S114 degree 2 poles (-15.0821, 7.3594) (-15.0568, 7.41) (-15.0234, 7.5407) (-15.0234, 7.6157) knots 0 0 0 1 2 2 2
  spline S115 degree 2 poles (-15.0234, 7.6157) (-15.0234, 7.796) (-15.2948, 8.0188) (-15.5207, 8.0188) knots 0 0 0 1 2 2 2
  spline S116 degree 2 poles (-15.5207, 8.0188) (-15.6463, 8.0188) (-15.8347, 7.9601) (-15.8996, 7.9044) knots 0 0 0 1 2 2 2
  spline S117 degree 2 poles (-15.8996, 7.9044) (-15.9644, 7.8507) (-16.0323, 7.6987) (-16.0323, 7.6035) knots 0 0 0 1 2 2 2
  spline S118 degree 2 poles (-16.0323, 7.6035) (-16.0323, 7.5336) (-16.012, 7.3938) (-15.9918, 7.3462) knots 0 0 0 1 2 2 2
  line L90 (-15.9918, 7.3462) -> (-15.6686, 7.3462)
  line L91 (-15.6686, 7.3462) -> (-15.6686, 7.6359)
  line L92 (-15.6686, 7.6359) -> (-15.5228, 7.6359)
  line L93 (-15.5228, 7.6359) -> (-15.5228, 7.1821)
  line L94 (-15.5228, 7.1821) -> (-16.0687, 7.1821)
  spline S119 degree 2 poles (-16.0687, 7.1821) (-16.0829, 7.2135) (-16.1265, 7.3209) (-16.1396, 7.3665) knots 0 0 0 1 2 2 2
  spline S120 degree 2 poles (-16.1396, 7.3665) (-16.1579, 7.4283) (-16.1761, 7.5275) (-16.1761, 7.5974) knots 0 0 0 1 2 2 2
  line L95 (-16.1518, 6.079) -> (-16.1518, 6.2654)
  line L96 (-16.1518, 6.2654) -> (-15.074, 6.8185)
  line L97 (-15.074, 6.8185) -> (-16.1518, 6.8185)
  line L98 (-16.1518, 6.8185) -> (-16.1518, 6.9734)
  line L99 (-16.1518, 6.9734) -> (-14.9018, 6.9734)
  line L100 (-14.9018, 6.9734) -> (-14.9018, 6.7374)
  line L101 (-14.9018, 6.7374) -> (-15.8915, 6.234)
  line L102 (-15.8915, 6.234) -> (-14.9018, 6.234)
  line L103 (-14.9018, 6.234) -> (-14.9018, 6.079)
  line L104 (-14.9018, 6.079) -> (-16.1518, 6.079)
  spline S121 degree 2 poles (-15.5278, 4.8401) (-15.699, 4.8401) (-15.9745, 4.9789) (-16.0515, 5.0954) knots 0 0 0 1 2 2 2
  spline S122 degree 2 poles (-16.0515, 5.0954) (-16.1113, 5.1906) (-16.1518, 5.3861) (-16.1518, 5.5381) knots 0 0 0 1 2 2 2
  line L105 (-16.1518, 5.5381) -> (-16.1518, 5.8258)
  line L106 (-16.1518, 5.8258) -> (-14.9018, 5.8258)
  line L107 (-14.9018, 5.8258) -> (-14.9018, 5.5411)
  spline S123 degree 2 poles (-14.9018, 5.5411) (-14.9018, 5.3649) (-14.9545, 5.1643) (-15.0011, 5.0934) knots 0 0 0 1 2 2 2
  spline S124 degree 2 poles (-15.0011, 5.0934) (-15.0811, 4.9728) (-15.3455, 4.8401) (-15.5278, 4.8401) knots 0 0 0 1 2 2 2
  spline S125 degree 2 poles (-15.5258, 5.0134) (-15.382, 5.0134) (-15.1783, 5.1086) (-15.1206, 5.2028) knots 0 0 0 1 2 2 2
  spline S126 degree 2 poles (-15.1206, 5.2028) (-15.0811, 5.2696) (-15.0456, 5.4206) (-15.0456, 5.533) knots 0 0 0 1 2 2 2
  line L108 (-15.0456, 5.533) -> (-15.0456, 5.6596)
  line L109 (-15.0456, 5.6596) -> (-16.008, 5.6596)
  line L110 (-16.008, 5.6596) -> (-16.008, 5.533)
  spline S127 degree 2 poles (-16.008, 5.533) (-16.008, 5.4226) (-15.9725, 5.2555) (-15.9249, 5.1876) knots 0 0 0 1 2 2 2
  spline S128 degree 2 poles (-15.9249, 5.1876) (-15.8661, 5.1005) (-15.6717, 5.0134) (-15.5258, 5.0134) knots 0 0 0 1 2 2 2
  spline S129 degree 2 poles (-15.0446, 3.2386) (-15.1277, 3.1677) (-15.3708, 3.0887) (-15.5268, 3.0887) knots 0 0 0 1 2 2 2
  spline S130 degree 2 poles (-15.5268, 3.0887) (-15.6787, 3.0887) (-15.9249, 3.1657) (-16.008, 3.2386) knots 0 0 0 1 2 2 2
  spline S131 degree 2 poles (-16.008, 3.2386) (-16.0951, 3.3156) (-16.1781, 3.5192) (-16.1781, 3.6418) knots 0 0 0 1 2 2 2
  spline S132 degree 2 poles (-16.1781, 3.6418) (-16.1781, 3.7684) (-16.092, 3.971) (-16.008, 4.045) knots 0 0 0 1 2 2 2
  spline S133 degree 2 poles (-16.008, 4.045) (-15.9249, 4.1169) (-15.6808, 4.1939) (-15.5268, 4.1939) knots 0 0 0 1 2 2 2
  spline S134 degree 2 poles (-15.5268, 4.1939) (-15.3698, 4.1939) (-15.1307, 4.1159) (-15.0446, 4.0439) knots 0 0 0 1 2 2 2
  spline S135 degree 2 poles (-15.0446, 4.0439) (-14.9616, 3.971) (-14.8755, 3.7674) (-14.8755, 3.6418) knots 0 0 0 1 2 2 2
  spline S136 degree 2 poles (-14.8755, 3.6418) (-14.8755, 3.5142) (-14.9646, 3.3095) (-15.0446, 3.2386) knots 0 0 0 1 2 2 2
  spline S137 degree 2 poles (-15.5268, 3.2619) (-15.4032, 3.2619) (-15.2118, 3.3156) (-15.149, 3.3642) knots 0 0 0 1 2 2 2
  spline S138 degree 2 poles (-15.149, 3.3642) (-15.0841, 3.4139) (-15.0193, 3.5537) (-15.0193, 3.6408) knots 0 0 0 1 2 2 2
  spline S139 degree 2 poles (-15.0193, 3.6408) (-15.0193, 3.7309) (-15.0821, 3.8667) (-15.149, 3.9183) knots 0 0 0 1 2 2 2
  spline S140 degree 2 poles (-15.149, 3.9183) (-15.2128, 3.968) (-15.4052, 4.0207) (-15.5268, 4.0207) knots 0 0 0 1 2 2 2
  spline S141 degree 2 poles (-15.5268, 4.0207) (-15.773, 4.0207) (-16.0343, 3.814) (-16.0343, 3.6408) knots 0 0 0 1 2 2 2
  spline S142 degree 2 poles (-16.0343, 3.6408) (-16.0343, 3.4676) (-15.773, 3.2619) (-15.5268, 3.2619) knots 0 0 0 1 2 2 2
  spline S143 degree 2 poles (-16.1781, 2.4698) (-16.1781, 2.5802) (-16.1204, 2.7443) (-16.0627, 2.8021) knots 0 0 0 1 2 2 2
  spline S144 degree 2 poles (-16.0627, 2.8021) (-15.9978, 2.8679) (-15.8155, 2.9216) (-15.6818, 2.9216) knots 0 0 0 1 2 2 2
  line L111 (-15.6818, 2.9216) -> (-14.9018, 2.9216)
  line L112 (-14.9018, 2.9216) -> (-14.9018, 2.7555)
  line L113 (-14.9018, 2.7555) -> (-15.6818, 2.7555)
  spline S145 degree 2 poles (-15.6818, 2.7555) (-15.7689, 2.7555) (-15.8864, 2.7332) (-15.934, 2.7018) knots 0 0 0 1 2 2 2
  spline S146 degree 2 poles (-15.934, 2.7018) (-15.9847, 2.6683) (-16.0363, 2.5529) (-16.0363, 2.4698) knots 0 0 0 1 2 2 2
  spline S147 degree 2 poles (-16.0363, 2.4698) (-16.0363, 2.3918) (-15.9847, 2.2702) (-15.934, 2.2368) knots 0 0 0 1 2 2 2
  spline S148 degree 2 poles (-15.934, 2.2368) (-15.8864, 2.2054) (-15.7699, 2.1831) (-15.6858, 2.1831) knots 0 0 0 1 2 2 2
  line L114 (-15.6858, 2.1831) -> (-14.9018, 2.1831)
  line L115 (-14.9018, 2.1831) -> (-14.9018, 2.017)
  line L116 (-14.9018, 2.017) -> (-15.6818, 2.017)
  spline S149 degree 2 poles (-15.6818, 2.017) (-15.8125, 2.017) (-15.9988, 2.0697) (-16.0627, 2.1365) knots 0 0 0 1 2 2 2
  spline S150 degree 2 poles (-16.0627, 2.1365) (-16.1214, 2.1963) (-16.1781, 2.3543) (-16.1781, 2.4698) knots 0 0 0 1 2 2 2
  line L117 (-16.1518, 1.4872) -> (-15.0497, 1.4872)
  line L118 (-15.0497, 1.4872) -> (-15.0497, 1.9066)
  line L119 (-15.0497, 1.9066) -> (-14.9018, 1.9066)
  line L120 (-14.9018, 1.9066) -> (-14.9018, 0.9017)
  line L121 (-14.9018, 0.9017) -> (-15.0497, 0.9017)
  line L122 (-15.0497, 0.9017) -> (-15.0497, 1.3211)
  line L123 (-15.0497, 1.3211) -> (-16.1518, 1.3211)
  line L124 (-16.1518, 1.3211) -> (-16.1518, 1.4872)
  spline S151 degree 2 poles (-16.1741, -0.1102) (-16.1741, 0.0255) (-16.1174, 0.216) (-16.0768, 0.3) knots 0 0 0 1 2 2 2
  line L125 (-16.0768, 0.3) -> (-15.8682, 0.3)
  line L126 (-15.8682, 0.3) -> (-15.8682, 0.2879)
  spline S152 degree 2 poles (-15.8682, 0.2879) (-15.9452, 0.2058) (-16.0302, -0.0018) (-16.0302, -0.0981) knots 0 0 0 1 2 2 2
  spline S153 degree 2 poles (-16.0302, -0.0981) (-16.0302, -0.2358) (-15.9158, -0.3766) (-15.8216, -0.3766) knots 0 0 0 1 2 2 2
  spline S154 degree 2 poles (-15.8216, -0.3766) (-15.7466, -0.3766) (-15.6534, -0.3027) (-15.6301, -0.2227) knots 0 0 0 1 2 2 2
  spline S155 degree 2 poles (-15.6301, -0.2227) (-15.6139, -0.1649) (-15.5916, -0.0687) (-15.5734, 0.0032) knots 0 0 0 1 2 2 2
  spline S156 degree 2 poles (-15.5734, 0.0032) (-15.5562, 0.0681) (-15.5045, 0.1704) (-15.463, 0.2099) knots 0 0 0 1 2 2 2
  spline S157 degree 2 poles (-15.463, 0.2099) (-15.4215, 0.2484) (-15.31, 0.2909) (-15.2371, 0.2909) knots 0 0 0 1 2 2 2
  spline S158 degree 2 poles (-15.2371, 0.2909) (-15.0852, 0.2909) (-14.8795, 0.0539) (-14.8795, -0.1295) knots 0 0 0 1 2 2 2
  spline S159 degree 2 poles (-14.8795, -0.1295) (-14.8795, -0.2348) (-14.9211, -0.4212) (-14.9606, -0.5012) knots 0 0 0 1 2 2 2
  line L127 (-14.9606, -0.5012) -> (-15.1591, -0.5012)
  line L128 (-15.1591, -0.5012) -> (-15.1591, -0.4891)
  spline S160 degree 2 poles (-15.1591, -0.4891) (-15.1044, -0.4293) (-15.0234, -0.2429) (-15.0234, -0.1406) knots 0 0 0 1 2 2 2
  spline S161 degree 2 poles (-15.0234, -0.1406) (-15.0234, -0.0251) (-15.1317, 0.1177) (-15.2199, 0.1177) knots 0 0 0 1 2 2 2
  spline S162 degree 2 poles (-15.2199, 0.1177) (-15.2989, 0.1177) (-15.3931, 0.0336) (-15.4144, -0.0454) knots 0 0 0 1 2 2 2
  spline S163 degree 2 poles (-15.4144, -0.0454) (-15.4285, -0.0981) (-15.465, -0.251) (-15.4802, -0.3017) knots 0 0 0 1 2 2 2
  spline S164 degree 2 poles (-15.4802, -0.3017) (-15.5197, -0.4303) (-15.6787, -0.5499) (-15.7952, -0.5499) knots 0 0 0 1 2 2 2
  spline S165 degree 2 poles (-15.7952, -0.5499) (-15.8692, -0.5499) (-16.011, -0.4901) (-16.0606, -0.4364) knots 0 0 0 1 2 2 2
  spline S166 degree 2 poles (-16.0606, -0.4364) (-16.1153, -0.3766) (-16.1741, -0.2247) (-16.1741, -0.1102) knots 0 0 0 1 2 2 2
  line L129 (-16.1518, -1.4544) -> (-16.1518, -0.6836)
  line L130 (-16.1518, -0.6836) -> (-15.9745, -0.6836)
  spline S167 degree 2 poles (-15.9745, -0.6836) (-15.8965, -0.7666) (-15.7517, -0.9145) (-15.6737, -0.9854) knots 0 0 0 1 2 2 2
  spline S168 degree 2 poles (-15.6737, -0.9854) (-15.5167, -1.1283) (-15.3283, -1.2326) (-15.228, -1.2326) knots 0 0 0 1 2 2 2
  spline S169 degree 2 poles (-15.228, -1.2326) (-15.1753, -1.2326) (-15.0963, -1.2002) (-15.071, -1.1708) knots 0 0 0 1 2 2 2
  spline S170 degree 2 poles (-15.071, -1.1708) (-15.0456, -1.1414) (-15.0203, -1.0644) (-15.0203, -1.0178) knots 0 0 0 1 2 2 2
  spline S171 degree 2 poles (-15.0203, -1.0178) (-15.0203, -0.9733) (-15.0426, -0.8821) (-15.0598, -0.8406) knots 0 0 0 1 2 2 2
  spline S172 degree 2 poles (-15.0598, -0.8406) (-15.074, -0.8051) (-15.1145, -0.7393) (-15.1287, -0.719) knots 0 0 0 1 2 2 2
  line L131 (-15.1287, -0.719) -> (-15.1287, -0.7099)
  line L132 (-15.1287, -0.7099) -> (-14.9504, -0.7099)
  spline S173 degree 2 poles (-14.9504, -0.7099) (-14.9251, -0.7616) (-14.8755, -0.9469) (-14.8755, -1.03) knots 0 0 0 1 2 2 2
  spline S174 degree 2 poles (-14.8755, -1.03) (-14.8755, -1.2052) (-15.0608, -1.4028) (-15.2189, -1.4028) knots 0 0 0 1 2 2 2
  spline S175 degree 2 poles (-15.2189, -1.4028) (-15.2928, -1.4028) (-15.4164, -1.3683) (-15.4691, -1.3379) knots 0 0 0 1 2 2 2
  spline S176 degree 2 poles (-15.4691, -1.3379) (-15.5238, -1.3075) (-15.6311, -1.2194) (-15.6828, -1.1708) knots 0 0 0 1 2 2 2
  spline S177 degree 2 poles (-15.6828, -1.1708) (-15.7689, -1.0918) (-15.9533, -0.8983) (-16.007, -0.8406) knots 0 0 0 1 2 2 2
  line L133 (-16.007, -0.8406) -> (-16.007, -1.4544)
  line L134 (-16.007, -1.4544) -> (-16.1518, -1.4544)
  spline S178 degree 2 poles (-16.1741, -2.5424) (-16.1741, -2.4066) (-16.1174, -2.2162) (-16.0768, -2.1321) knots 0 0 0 1 2 2 2
  line L135 (-16.0768, -2.1321) -> (-15.8682, -2.1321)
  line L136 (-15.8682, -2.1321) -> (-15.8682, -2.1443)
  spline S179 degree 2 poles (-15.8682, -2.1443) (-15.9452, -2.2263) (-16.0302, -2.434) (-16.0302, -2.5302) knots 0 0 0 1 2 2 2
  spline S180 degree 2 poles (-16.0302, -2.5302) (-16.0302, -2.668) (-15.9158, -2.8088) (-15.8216, -2.8088) knots 0 0 0 1 2 2 2
  spline S181 degree 2 poles (-15.8216, -2.8088) (-15.7466, -2.8088) (-15.6534, -2.7348) (-15.6301, -2.6548) knots 0 0 0 1 2 2 2
  spline S182 degree 2 poles (-15.6301, -2.6548) (-15.6139, -2.5971) (-15.5916, -2.5008) (-15.5734, -2.4289) knots 0 0 0 1 2 2 2
  spline S183 degree 2 poles (-15.5734, -2.4289) (-15.5562, -2.3641) (-15.5045, -2.2618) (-15.463, -2.2223) knots 0 0 0 1 2 2 2
  spline S184 degree 2 poles (-15.463, -2.2223) (-15.4215, -2.1838) (-15.31, -2.1412) (-15.2371, -2.1412) knots 0 0 0 1 2 2 2
  spline S185 degree 2 poles (-15.2371, -2.1412) (-15.0852, -2.1412) (-14.8795, -2.3783) (-14.8795, -2.5616) knots 0 0 0 1 2 2 2
  spline S186 degree 2 poles (-14.8795, -2.5616) (-14.8795, -2.6669) (-14.9211, -2.8533) (-14.9606, -2.9334) knots 0 0 0 1 2 2 2
  line L137 (-14.9606, -2.9334) -> (-15.1591, -2.9334)
  line L138 (-15.1591, -2.9334) -> (-15.1591, -2.9212)
  spline S187 degree 2 poles (-15.1591, -2.9212) (-15.1044, -2.8614) (-15.0234, -2.6751) (-15.0234, -2.5727) knots 0 0 0 1 2 2 2
  spline S188 degree 2 poles (-15.0234, -2.5727) (-15.0234, -2.4573) (-15.1317, -2.3144) (-15.2199, -2.3144) knots 0 0 0 1 2 2 2
  spline S189 degree 2 poles (-15.2199, -2.3144) (-15.2989, -2.3144) (-15.3931, -2.3985) (-15.4144, -2.4775) knots 0 0 0 1 2 2 2
  spline S190 degree 2 poles (-15.4144, -2.4775) (-15.4285, -2.5302) (-15.465, -2.6832) (-15.4802, -2.7338) knots 0 0 0 1 2 2 2
  spline S191 degree 2 poles (-15.4802, -2.7338) (-15.5197, -2.8625) (-15.6787, -2.982) (-15.7952, -2.982) knots 0 0 0 1 2 2 2
  spline S192 degree 2 poles (-15.7952, -2.982) (-15.8692, -2.982) (-16.011, -2.9222) (-16.0606, -2.8685) knots 0 0 0 1 2 2 2
  spline S193 degree 2 poles (-16.0606, -2.8685) (-16.1153, -2.8088) (-16.1741, -2.6568) (-16.1741, -2.5424) knots 0 0 0 1 2 2 2
  spline S194 degree 2 poles (-15.0203, -3.453) (-15.0203, -3.4074) (-15.0426, -3.3173) (-15.0598, -3.2737) knots 0 0 0 1 2 2 2
  spline S195 degree 2 poles (-15.0598, -3.2737) (-15.077, -3.2332) (-15.1135, -3.1734) (-15.1297, -3.1501) knots 0 0 0 1 2 2 2
  line L139 (-15.1297, -3.1501) -> (-15.1297, -3.14)
  line L140 (-15.1297, -3.14) -> (-14.9525, -3.14)
  spline S196 degree 2 poles (-14.9525, -3.14) (-14.9231, -3.1947) (-14.8755, -3.3821) (-14.8755, -3.4662) knots 0 0 0 1 2 2 2
  spline S197 degree 2 poles (-14.8755, -3.4662) (-14.8755, -3.5513) (-14.9099, -3.6779) (-14.9464, -3.7296) knots 0 0 0 1 2 2 2
  spline S198 degree 2 poles (-14.9464, -3.7296) (-14.9859, -3.7843) (-15.1003, -3.841) (-15.1773, -3.841) knots 0 0 0 1 2 2 2
  spline S199 degree 2 poles (-15.1773, -3.841) (-15.2807, -3.841) (-15.4367, -3.7052) (-15.4569, -3.61) knots 0 0 0 1 2 2 2
  line L141 (-15.4569, -3.61) -> (-15.4691, -3.61)
  spline S200 degree 2 poles (-15.4691, -3.61) (-15.4772, -3.6495) (-15.5136, -3.7397) (-15.5501, -3.7782) knots 0 0 0 1 2 2 2
  spline S201 degree 2 poles (-15.5501, -3.7782) (-15.5856, -3.8167) (-15.699, -3.8653) (-15.7811, -3.8653) knots 0 0 0 1 2 2 2
  spline S202 degree 2 poles (-15.7811, -3.8653) (-15.8651, -3.8653) (-16.008, -3.8075) (-16.0627, -3.7549) knots 0 0 0 1 2 2 2
  spline S203 degree 2 poles (-16.0627, -3.7549) (-16.1194, -3.7002) (-16.1781, -3.5452) (-16.1781, -3.4469) knots 0 0 0 1 2 2 2
  spline S204 degree 2 poles (-16.1781, -3.4469) (-16.1781, -3.3527) (-16.1326, -3.1684) (-16.1012, -3.1056) knots 0 0 0 1 2 2 2
  line L142 (-16.1012, -3.1056) -> (-15.9239, -3.1056)
  line L143 (-15.9239, -3.1056) -> (-15.9239, -3.1177)
  spline S205 degree 2 poles (-15.9239, -3.1177) (-15.9624, -3.1704) (-16.0333, -3.3487) (-16.0333, -3.4368) knots 0 0 0 1 2 2 2
  spline S206 degree 2 poles (-16.0333, -3.4368) (-16.0333, -3.4885) (-16.0009, -3.5918) (-15.9634, -3.6262) knots 0 0 0 1 2 2 2
  spline S207 degree 2 poles (-15.9634, -3.6262) (-15.9259, -3.6597) (-15.8368, -3.6951) (-15.7689, -3.6951) knots 0 0 0 1 2 2 2
  spline S208 degree 2 poles (-15.7689, -3.6951) (-15.701, -3.6951) (-15.6129, -3.6556) (-15.5876, -3.6202) knots 0 0 0 1 2 2 2
  spline S209 degree 2 poles (-15.5876, -3.6202) (-15.5623, -3.5847) (-15.543, -3.4885) (-15.543, -3.4317) knots 0 0 0 1 2 2 2
  line L144 (-15.543, -3.4317) -> (-15.543, -3.3608)
  line L145 (-15.543, -3.3608) -> (-15.4042, -3.3608)
  line L146 (-15.4042, -3.3608) -> (-15.4042, -3.4165)
  spline S210 degree 2 poles (-15.4042, -3.4165) (-15.4042, -3.529) (-15.2969, -3.6708) (-15.1946, -3.6708) knots 0 0 0 1 2 2 2
  spline S211 degree 2 poles (-15.1946, -3.6708) (-15.1469, -3.6708) (-15.0791, -3.6343) (-15.0588, -3.605) knots 0 0 0 1 2 2 2
  spline S212 degree 2 poles (-15.0588, -3.605) (-15.0375, -3.5736) (-15.0203, -3.4966) (-15.0203, -3.453) knots 0 0 0 1 2 2 2
  line L147 (-14.9018, -5.5326) -> (-16.1518, -5.1021)
  line L148 (-16.1518, -5.1021) -> (-16.1518, -4.9228)
  line L149 (-16.1518, -4.9228) -> (-14.9018, -4.4923)
  line L150 (-14.9018, -4.4923) -> (-14.9018, -4.6706)
  line L151 (-14.9018, -4.6706) -> (-15.9401, -5.017)
  line L152 (-15.9401, -5.017) -> (-14.9018, -5.3635)
  line L153 (-14.9018, -5.3635) -> (-14.9018, -5.5326)
  spline S213 degree 2 poles (-16.1741, -6.1404) (-16.1741, -6.0189) (-16.092, -5.8132) (-16.01, -5.7383) knots 0 0 0 1 2 2 2
  spline S214 degree 2 poles (-16.01, -5.7383) (-15.929, -5.6633) (-15.6858, -5.5813) (-15.5278, -5.5813) knots 0 0 0 1 2 2 2
  spline S215 degree 2 poles (-15.5278, -5.5813) (-15.3708, -5.5813) (-15.1378, -5.6613) (-15.0517, -5.7372) knots 0 0 0 1 2 2 2
  spline S216 degree 2 poles (-15.0517, -5.7372) (-14.9676, -5.8122) (-14.8795, -6.0168) (-14.8795, -6.1434) knots 0 0 0 1 2 2 2
  spline S217 degree 2 poles (-14.8795, -6.1434) (-14.8795, -6.2063) (-14.8978, -6.3167) (-14.9119, -6.3633) knots 0 0 0 1 2 2 2
  spline S218 degree 2 poles (-14.9119, -6.3633) (-14.9251, -6.4038) (-14.9626, -6.4879) (-14.9849, -6.5294) knots 0 0 0 1 2 2 2
  line L154 (-14.9849, -6.5294) -> (-15.1854, -6.5294)
  line L155 (-15.1854, -6.5294) -> (-15.1854, -6.5162)
  spline S219 degree 2 poles (-15.1854, -6.5162) (-15.1652, -6.4939) (-15.1084, -6.4251) (-15.0811, -6.3754) knots 0 0 0 1 2 2 2
  spline S220 degree 2 poles (-15.0811, -6.3754) (-15.0548, -6.3278) (-15.0213, -6.2154) (-15.0213, -6.1424) knots 0 0 0 1 2 2 2
  spline S221 degree 2 poles (-15.0213, -6.1424) (-15.0213, -6.0624) (-15.0872, -5.9196) (-15.15, -5.8659) knots 0 0 0 1 2 2 2
  spline S222 degree 2 poles (-15.15, -5.8659) (-15.2138, -5.8132) (-15.4073, -5.7545) (-15.5278, -5.7545) knots 0 0 0 1 2 2 2
  spline S223 degree 2 poles (-15.5278, -5.7545) (-15.6565, -5.7545) (-15.8418, -5.8163) (-15.9057, -5.8699) knots 0 0 0 1 2 2 2
  spline S224 degree 2 poles (-15.9057, -5.8699) (-15.9674, -5.9226) (-16.0302, -6.0634) (-16.0302, -6.1424) knots 0 0 0 1 2 2 2
  spline S225 degree 2 poles (-16.0302, -6.1424) (-16.0302, -6.2144) (-15.9948, -6.3369) (-15.9685, -6.3845) knots 0 0 0 1 2 2 2
  spline S226 degree 2 poles (-15.9685, -6.3845) (-15.9421, -6.4301) (-15.8874, -6.498) (-15.8682, -6.5172) knots 0 0 0 1 2 2 2
  line L156 (-15.8682, -6.5172) -> (-15.8682, -6.5294)
  line L157 (-15.8682, -6.5294) -> (-16.0667, -6.5294)
  spline S227 degree 2 poles (-16.0667, -6.5294) (-16.086, -6.4879) (-16.1214, -6.4149) (-16.1376, -6.3633) knots 0 0 0 1 2 2 2
  spline S228 degree 2 poles (-16.1376, -6.3633) (-16.1559, -6.3086) (-16.1741, -6.2154) (-16.1741, -6.1404) knots 0 0 0 1 2 2 2
  spline S229 degree 2 poles (-16.1741, -7.1726) (-16.1741, -7.0511) (-16.092, -6.8454) (-16.01, -6.7705) knots 0 0 0 1 2 2 2
  spline S230 degree 2 poles (-16.01, -6.7705) (-15.929, -6.6955) (-15.6858, -6.6135) (-15.5278, -6.6135) knots 0 0 0 1 2 2 2
  spline S231 degree 2 poles (-15.5278, -6.6135) (-15.3708, -6.6135) (-15.1378, -6.6935) (-15.0517, -6.7695) knots 0 0 0 1 2 2 2
  spline S232 degree 2 poles (-15.0517, -6.7695) (-14.9676, -6.8444) (-14.8795, -7.049) (-14.8795, -7.1757) knots 0 0 0 1 2 2 2
  spline S233 degree 2 poles (-14.8795, -7.1757) (-14.8795, -7.2385) (-14.8978, -7.3489) (-14.9119, -7.3955) knots 0 0 0 1 2 2 2
  spline S234 degree 2 poles (-14.9119, -7.3955) (-14.9251, -7.436) (-14.9626, -7.5201) (-14.9849, -7.5616) knots 0 0 0 1 2 2 2
  line L158 (-14.9849, -7.5616) -> (-15.1854, -7.5616)
  line L159 (-15.1854, -7.5616) -> (-15.1854, -7.5484)
  spline S235 degree 2 poles (-15.1854, -7.5484) (-15.1652, -7.5261) (-15.1084, -7.4573) (-15.0811, -7.4076) knots 0 0 0 1 2 2 2
  spline S236 degree 2 poles (-15.0811, -7.4076) (-15.0548, -7.36) (-15.0213, -7.2476) (-15.0213, -7.1746) knots 0 0 0 1 2 2 2
  spline S237 degree 2 poles (-15.0213, -7.1746) (-15.0213, -7.0946) (-15.0872, -6.9518) (-15.15, -6.8981) knots 0 0 0 1 2 2 2
  spline S238 degree 2 poles (-15.15, -6.8981) (-15.2138, -6.8454) (-15.4073, -6.7867) (-15.5278, -6.7867) knots 0 0 0 1 2 2 2
  spline S239 degree 2 poles (-15.5278, -6.7867) (-15.6565, -6.7867) (-15.8418, -6.8485) (-15.9057, -6.9022) knots 0 0 0 1 2 2 2
  spline S240 degree 2 poles (-15.9057, -6.9022) (-15.9674, -6.9548) (-16.0302, -7.0956) (-16.0302, -7.1746) knots 0 0 0 1 2 2 2
  spline S241 degree 2 poles (-16.0302, -7.1746) (-16.0302, -7.2466) (-15.9948, -7.3691) (-15.9685, -7.4167) knots 0 0 0 1 2 2 2
  spline S242 degree 2 poles (-15.9685, -7.4167) (-15.9421, -7.4623) (-15.8874, -7.5302) (-15.8682, -7.5494) knots 0 0 0 1 2 2 2
  line L160 (-15.8682, -7.5494) -> (-15.8682, -7.5616)
  line L161 (-15.8682, -7.5616) -> (-16.0667, -7.5616)
  spline S243 degree 2 poles (-16.0667, -7.5616) (-16.086, -7.5201) (-16.1214, -7.4471) (-16.1376, -7.3955) knots 0 0 0 1 2 2 2
  spline S244 degree 2 poles (-16.1376, -7.3955) (-16.1559, -7.3408) (-16.1741, -7.2476) (-16.1741, -7.1726) knots 0 0 0 1 2 2 2
  point P0 (0, 0)
  constraints: 4 other
extrude "Extrusion6" add sketch "Sketch8" along normal blind 0.01